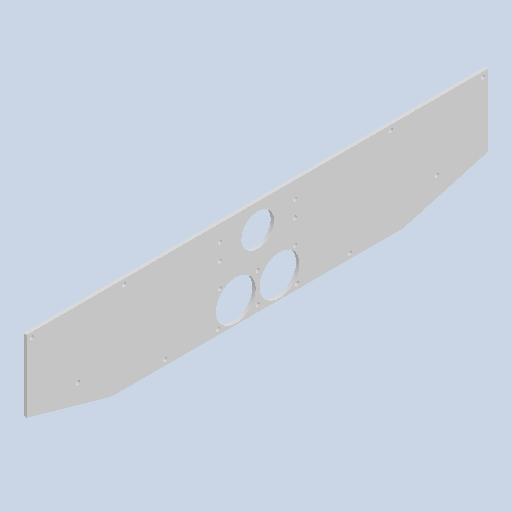
# Autodesk Inventor part: insideChassiPlate2.0
Saved by Autodesk Inventor 2023 (Build 270158000, 158)
## iProperties
Created: 2022-09-08
Part Number: insideChassiPlate2.0
Material: Generic
Document SubType Name: Modeling
Designer: deli
Density: 1 g/cm^3
Appearance: Default
Author: deli
Autodesk Inventor part; units mm, degrees
ref_plane "YZ Plane" through (0, 0, 0) normal (1, 0, 0) x (0, 1, 0)
ref_plane "XZ Plane" through (0, 0, 0) normal (0, 1, 0) x (-1, 0, 0)
ref_plane "XY Plane" through (0, 0, 0) normal (0, 0, 1) x (1, 0, 0)
sketch "Sketch1" plane through (0, 0, 0) normal (1, 0, 0) x (0, 1, 0)
  line L0 (-34.0027, 86.5738) -> (-104.0027, 86.5738)
  line L1 (-104.0027, 86.5738) -> (-127.2253, 4.3058)
  arc A0 (-127.2253, 4.3058) -> (-127.4133, 2.9475) centre (-122.4133, 2.9475) ccw
  line L2 (-127.4133, 2.9475) -> (-127.4133, -279.7999)
  arc A1 (-127.4133, -279.7999) -> (-127.2253, -281.1582) centre (-122.4133, -279.7999) ccw
  line L3 (-127.2253, -281.1582) -> (-104.0027, -363.4262)
  line L4 (-104.0027, -363.4262) -> (-34.0027, -363.4262)
  line L5 (-34.0027, -363.4262) -> (-34.0027, -226.9762)
  line L6 (-34.0027, -226.9762) -> (230.9973, -226.9762)
  line L7 (230.9973, -226.9762) -> (230.9973, -201.5762)
  line L8 (230.9973, -201.5762) -> (-34.0027, -201.5762)
  line L9 (-34.0027, -201.5762) -> (-34.0027, 86.5738)
  circle A2 centre (-66.0027, -101.9662) radius 2
  circle A3 centre (-122.4133, -228.31) radius 2
  circle A4 centre (-122.4133, -48.5424) radius 2
  circle A5 centre (-39.0027, -8.4262) radius 2
  circle A6 centre (-39.0027, -358.4262) radius 2
  circle A7 centre (-89.2685, -175.1441) radius 2
  circle A8 centre (-99.4133, 36.5738) radius 2
  circle A9 centre (-99.4133, -313.4262) radius 2
  circle A10 centre (-106.6633, -117.135) radius 7 construction
  circle A11 centre (-106.6633, -159.7175) radius 7 construction
  circle A12 centre (-92.1807, -138.4262) radius 2
  circle A13 centre (-121.1459, -138.4262) radius 2
  circle A14 centre (-122.4133, -100.0323) radius 2
  circle A15 centre (-122.4133, -176.8201) radius 2
  circle A16 centre (-39.0027, 81.5738) radius 2
  circle A17 centre (-89.2685, -101.7083) radius 2
  circle A18 centre (-39.0027, -268.4262) radius 2
  circle A19 centre (222.9973, -212.6887) radius 2
  circle A20 centre (-58.0027, -138.4262) radius 16
  circle A21 centre (-50.0027, -101.9662) radius 2
  line L10 (-34.0027, -201.5762) -> (-34.0027, -226.9762)
  spline S0 degree 3 number of poles 284
  spline S1 degree 3 number of poles 284
  circle A22 centre (-50.0027, -174.8862) radius 2
  circle A23 centre (-66.0027, -174.8862) radius 2
  circle A24 centre (-66.0027, -174.8862) radius 2
  circle A25 centre (-50.0027, -174.8862) radius 2
  line L11 (-50.0027, -101.9662) -> (-66.0027, -101.9662) construction
  line L12 (-66.0027, -101.9662) -> (-66.0027, -174.8862) construction
  line L13 (-66.0027, -174.8862) -> (-50.0027, -174.8862) construction
  line L14 (-50.0027, -174.8862) -> (-50.0027, -101.9662) construction
  circle A26 centre (-106.6633, -117.135) radius 19.5
  circle A27 centre (-106.6633, -159.7175) radius 19.5
  dimension "d6" = 4
  dimension "d7" = 4
  dimension "d8" = 39
  dimension "d9" = 39
  constraints: 10 end point, 4 centre point, 4 coincident, 2 parallel, 1 horizontal, 1 perpendicular, 1 vertical
  measures "d6" diameter of A24
  measures "d7" diameter of A25
  measures "d8" diameter of A26
  measures "d9" diameter of A27
extrude "Extrusion1" add sketch "Sketch1" along normal blind 3.175 contours L9 L10 L5 L4 L3 A1 L2 A0 L1 L0
body "Solid1"
